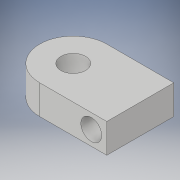
# Autodesk Inventor part: Bearing O
Saved by Autodesk Inventor 2018 (Build 220112000, 112)
## iProperties
Created: 2018-01-15
Part Number: Bearing O
Material: Generic
Document SubType Name: Modeling
Designer: junai
Density: 1 g/cm^3
Appearance: Default
Author: junai
Autodesk Inventor part; units mm, degrees
ref_plane "YZ Plane" through (0, 0, 0) normal (1, 0, 0) x (0, 1, 0)
ref_plane "XZ Plane" through (0, 0, 0) normal (0, 1, 0) x (-1, 0, 0)
ref_plane "XY Plane" through (0, 0, 0) normal (0, 0, 1) x (1, 0, 0)
sketch "Sketch1" plane through (0, 0, 0) normal (0, 1, 0) x (-1, 0, 0)
  line L0 (11, 8) -> (-11, 8)
  line L1 (-11, 8) -> (-11, -8)
  line L2 (-11, -8) -> (11, -8)
  line L3 (11, -8) -> (11, 8)
  line L4 (0, 0) -> (0, -8) construction
  line L5 (0, 0) -> (11, 0) construction
  dimension "d0" = 16
  dimension "d1" = 22
  dimension "d2" = 8
  dimension "d3" = 11
  constraints: 12 end point, 2 horizontal, 2 midpoint, 2 parallel, 2 perpendicular, 1 vertical
  measures "d0" distance of L0.end L1.end
  measures "d1" distance of L1.end L2.end
  measures "d2" distance of L4.start L4.end
  measures "d3" distance of L4.start L5.end
extrude "Extrusion1" add sketch "Sketch1" along normal blind 9.6
sketch "Sketch2" plane through (-11, 0, 8) normal (0, 0, 1) x (1, 0, 0)
  line L0 (22, 0) -> (22, 9.6) projected
  line L1 (22, 4.8) -> (16.92, 4.8) construction
  circle A0 centre (16.92, 4.8) radius 3.425
  point P0 (11, 0)
  dimension "d6" = 5.08
  dimension "d8" = 6.85
  constraints: 2 end point, 1 centre point, 1 coincident, 1 horizontal, 1 midpoint
  measures "d6" distance of L1.start L1.end
  measures "d8" diameter of A0
sketch "Sketch3" plane through (-11, 0, -8) normal (-1, 0, 0) x (0, 0, 1)
  point P0 (8, 0)
sketch "Sketch4" plane through (0, 9.6, 0) normal (0, 1, 0) x (1, 0, 0)
  line L0 (-11, 8) -> (-11, -8) projected
  line L1 (11, -8) -> (-11, -8)
  line L2 (-11, -8) -> (-11, 14)
  line L3 (-11, 14) -> (11, 14)
  line L4 (11, 14) -> (11, -8)
  point P0 (0, 0)
  dimension "d10" = 22
  constraints: 8 end point, 2 parallel, 1 horizontal, 1 perpendicular
  measures "d10" distance of L3.end L1.start
extrude "Extrusion2" add sketch "Sketch4" against normal blind 9.6
sketch "Sketch5" plane through (0, 9.6, 0) normal (0, 1, 0) x (1, 0, 0)
  line L0 (-11, -8) -> (-11, 14) projected
  circle A0 centre (-11, 3) radius 11
  point P0 (0, 0)
  constraints: 1 midpoint, 1 vertical alignment, 2 other
extrude "Extrusion3" add sketch "Sketch5" against normal blind 9.6
extrude "Extrusion4" cut sketch "Sketch2" against normal through all
sketch "Sketch6" plane through (0, 9.6, 0) normal (0, 1, 0) x (1, 0, 0)
  circle A0 centre (-11, 3) radius 6.35
  arc A1 (-11, 14) -> (-11, -8) centre (-11, 3) ccw projected
  point P0 (0, 0)
  dimension "d17" = 12.7
  constraints: 1 centre point, 1 concentric
  measures "d17" diameter of A0
extrude "Extrusion5" cut sketch "Sketch6" against normal up to next
sketch "Sketch7" plane through (0, 9.6, 0) normal (0, 1, 0) x (1, 0, 0)
  circle A0 centre (-11, 3) radius 6.35 projected
  circle A1 centre (-11, 3) radius 6.35
  circle A2 centre (-11, 3) radius 4.05
  point P0 (0, 0)
  dimension "d20" = 8.1
  constraints: 2 centre point, 2 coincident, 1 concentric
  measures "d20" diameter of A2
extrude "Extrusion6" add sketch "Sketch7" against normal up to surface (9.6 mm away)
equation "\"d18\" = d17"
body "Solid1"
